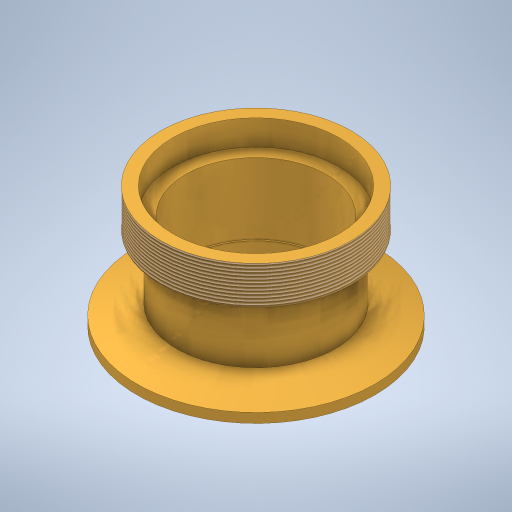
# Autodesk Inventor part: KF_fitting
Saved by Autodesk Inventor 2024 (Build 280153000, 153)
## iProperties
Created: 2023-11-04
Part Number: KF_fitting
Material: Brass, Soft Yellow
Document SubType Name: Modeling
Designer: schanen
Density: 8.47 g/cm^3
Appearance: Brass - Satin
neck_thread_dia: 30.000 mm
neck_thread_len: 12.000 mm
neck_ir: 22.225 mm
Author: schanen
Autodesk Inventor part; units mm, degrees
ref_plane "YZ Plane" through (0, 0, 0) normal (1, 0, 0) x (0, 1, 0)
ref_plane "XZ Plane" through (0, 0, 0) normal (0, 1, 0) x (-1, 0, 0)
ref_plane "XY Plane" through (0, 0, 0) normal (0, 0, 1) x (1, 0, 0)
sketch "Sketch1" plane through (0, 0, 0) normal (0, 0, 1) x (1, 0, 0)
  line L0 (-22.225, 22.3494) -> (-22.225, 0)
  line L1 (-25, -1.6506) -> (-25, 18.3494)
  line L2 (-25, 18.3494) -> (-30, 18.3494)
  line L3 (-30, 18.3494) -> (-30, 30.3494)
  line L4 (-30, 30.3494) -> (-26.225, 30.3494)
  line L5 (-26.225, 30.3494) -> (-26.225, 22.3494)
  line L6 (-26.225, 22.3494) -> (-22.225, 22.3494)
  line L7 (0, -15.6699) -> (0, 38.0192) projected
  line L8 (-25, -1.6506) -> (-37.5, -5)
  line L9 (-37.5, -5) -> (-37.5, -8)
  line L10 (-37.5, -8) -> (-26, -8)
  line L11 (-26, -8) -> (-26, -5)
  line L12 (-26, -5) -> (-21.725, -5)
  line L13 (-21.725, -5) -> (-21.725, 0)
  line L14 (-21.725, 0) -> (-22.225, 0)
  point P0 (0, 0)
  dimension "neck_ir" = 22.225
  dimension "d3" = 4
  dimension "d4" = 8
  dimension "neck_thread_dia" = 30
  dimension "neck_thread_len" = 12
  dimension "d14" = 26
  dimension "d15" = 21.725
  dimension "d16" = 3
  dimension "d17" = 15
  dimension "d18" = 3
  dimension "d19" = 37.5
  dimension "d20" = 25
  dimension "d21" = 20
  dimension "d22" = 5
  constraints: 28 end point, 9 perpendicular, 2 vertical, 1 horizontal, 1 horizontal alignment
  measures "neck_ir" distance from line of point (0, 0) L0
  measures "d3" distance of L5.end L0.start
  measures "d4" distance of L4.end L5.end
  measures "neck_thread_dia" distance from line of point (0, 0) L3
  measures "neck_thread_len" distance of L2.end L3.end
  measures "d14" distance between parallel lines of L7 L11
  measures "d15" distance between parallel lines of L7 L13
  measures "d16" distance of L8.end L9.end
  measures "d17" angle of L8 L10
  measures "d18" distance of L10.end L11.end
  measures "d19" distance between parallel lines of L7 L9
  measures "d20" distance between parallel lines of L7 L1
  measures "d21" distance of L1.start L1.end
  measures "d22" distance of L12.end L13.end
revolve "Revolution1" add sketch "Sketch1" angle 360 about axis through (0, -10, 0) along (0, 1, 0)
thread "Thread1" size "M60x1" class "6g" standard "ANSI Metric M Profile" full length
equation "\"neck_ir\" = 0.5 * cylinder_od"
equation "\"d3\" = oring_diameter"
equation "\"d4\" = 2 * oring_diameter"
equation "\"d15\" = 0.5 * cylinder_od - cylinder_wall"
equation "\"oring_diameter\" = 4"
equation "\"cylinder_od\" = 44.45"
equation "\"cylinder_wall\" = 0.5"
body "Solid1"
